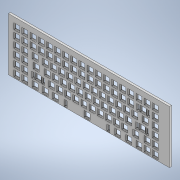
# Autodesk Inventor part: Top Plate
Saved by Autodesk Inventor 2020 (Build 240168000, 168)
## iProperties
Created: 2019-09-30
Part Number: Top Plate
Material: Generic
Document SubType Name: Sheet Metal
Designer: risha
Density: 1 g/cm^3
Sheet Metal Rule: Default_mm
Appearance: Default
Author: risha
Autodesk Inventor part; units mm, degrees
(part 1 of 2)
ref_plane "YZ Plane" through (0, 0, 0) normal (1, 0, 0) x (0, 1, 0)
ref_plane "XZ Plane" through (0, 0, 0) normal (0, 1, 0) x (-1, 0, 0)
ref_plane "XY Plane" through (0, 0, 0) normal (0, 0, 1) x (1, 0, 0)
sketch "Sketch1" plane through (0, 0, 0) normal (0, 0, 1) x (1, 0, 0)
  line L0 (3.025, -2.525) -> (16.025, -2.525)
  line L1 (3.025, -16.525) -> (16.025, -16.525)
  line L2 (2.525, -3.025) -> (2.525, -16.025)
  line L3 (16.525, -3.025) -> (16.525, -16.025)
  arc A0 (3.025, -2.525) -> (2.525, -3.025) centre (3.025, -3.025) ccw
  arc A1 (16.525, -3.025) -> (16.025, -2.525) centre (16.025, -3.025) ccw
  arc A2 (2.525, -16.025) -> (3.025, -16.525) centre (3.025, -16.025) ccw
  arc A3 (16.025, -16.525) -> (16.525, -16.025) centre (16.025, -16.025) ccw
  line L4 (22.075, -2.525) -> (35.075, -2.525)
  line L5 (22.075, -16.525) -> (35.075, -16.525)
  line L6 (21.575, -3.025) -> (21.575, -16.025)
  line L7 (35.575, -3.025) -> (35.575, -16.025)
  arc A4 (22.075, -2.525) -> (21.575, -3.025) centre (22.075, -3.025) ccw
  arc A5 (35.575, -3.025) -> (35.075, -2.525) centre (35.075, -3.025) ccw
  arc A6 (21.575, -16.025) -> (22.075, -16.525) centre (22.075, -16.025) ccw
  arc A7 (35.075, -16.525) -> (35.575, -16.025) centre (35.075, -16.025) ccw
  line L8 (41.125, -2.525) -> (54.125, -2.525)
  line L9 (41.125, -16.525) -> (54.125, -16.525)
  line L10 (40.625, -3.025) -> (40.625, -16.025)
  line L11 (54.625, -3.025) -> (54.625, -16.025)
  arc A8 (41.125, -2.525) -> (40.625, -3.025) centre (41.125, -3.025) ccw
  arc A9 (54.625, -3.025) -> (54.125, -2.525) centre (54.125, -3.025) ccw
  arc A10 (40.625, -16.025) -> (41.125, -16.525) centre (41.125, -16.025) ccw
  arc A11 (54.125, -16.525) -> (54.625, -16.025) centre (54.125, -16.025) ccw
  line L12 (60.175, -2.525) -> (73.175, -2.525)
  line L13 (60.175, -16.525) -> (73.175, -16.525)
  line L14 (59.675, -3.025) -> (59.675, -16.025)
  line L15 (73.675, -3.025) -> (73.675, -16.025)
  arc A12 (60.175, -2.525) -> (59.675, -3.025) centre (60.175, -3.025) ccw
  arc A13 (73.675, -3.025) -> (73.175, -2.525) centre (73.175, -3.025) ccw
  arc A14 (59.675, -16.025) -> (60.175, -16.525) centre (60.175, -16.025) ccw
  arc A15 (73.175, -16.525) -> (73.675, -16.025) centre (73.175, -16.025) ccw
  line L16 (79.225, -2.525) -> (92.225, -2.525)
  line L17 (79.225, -16.525) -> (92.225, -16.525)
  line L18 (78.725, -3.025) -> (78.725, -16.025)
  line L19 (92.725, -3.025) -> (92.725, -16.025)
  arc A16 (79.225, -2.525) -> (78.725, -3.025) centre (79.225, -3.025) ccw
  arc A17 (92.725, -3.025) -> (92.225, -2.525) centre (92.225, -3.025) ccw
  arc A18 (78.725, -16.025) -> (79.225, -16.525) centre (79.225, -16.025) ccw
  arc A19 (92.225, -16.525) -> (92.725, -16.025) centre (92.225, -16.025) ccw
  line L20 (98.275, -2.525) -> (111.275, -2.525)
  line L21 (98.275, -16.525) -> (111.275, -16.525)
  line L22 (97.775, -3.025) -> (97.775, -16.025)
  line L23 (111.775, -3.025) -> (111.775, -16.025)
  arc A20 (98.275, -2.525) -> (97.775, -3.025) centre (98.275, -3.025) ccw
  arc A21 (111.775, -3.025) -> (111.275, -2.525) centre (111.275, -3.025) ccw
  arc A22 (97.775, -16.025) -> (98.275, -16.525) centre (98.275, -16.025) ccw
  arc A23 (111.275, -16.525) -> (111.775, -16.025) centre (111.275, -16.025) ccw
  line L24 (117.325, -2.525) -> (130.325, -2.525)
  line L25 (117.325, -16.525) -> (130.325, -16.525)
  line L26 (116.825, -3.025) -> (116.825, -16.025)
  line L27 (130.825, -3.025) -> (130.825, -16.025)
  arc A24 (117.325, -2.525) -> (116.825, -3.025) centre (117.325, -3.025) ccw
  arc A25 (130.825, -3.025) -> (130.325, -2.525) centre (130.325, -3.025) ccw
  arc A26 (116.825, -16.025) -> (117.325, -16.525) centre (117.325, -16.025) ccw
  arc A27 (130.325, -16.525) -> (130.825, -16.025) centre (130.325, -16.025) ccw
  line L28 (136.375, -2.525) -> (149.375, -2.525)
  line L29 (136.375, -16.525) -> (149.375, -16.525)
  line L30 (135.875, -3.025) -> (135.875, -16.025)
  line L31 (149.875, -3.025) -> (149.875, -16.025)
  arc A28 (136.375, -2.525) -> (135.875, -3.025) centre (136.375, -3.025) ccw
  arc A29 (149.875, -3.025) -> (149.375, -2.525) centre (149.375, -3.025) ccw
  arc A30 (135.875, -16.025) -> (136.375, -16.525) centre (136.375, -16.025) ccw
  arc A31 (149.375, -16.525) -> (149.875, -16.025) centre (149.375, -16.025) ccw
  line L32 (155.425, -2.525) -> (168.425, -2.525)
  line L33 (155.425, -16.525) -> (168.425, -16.525)
  line L34 (154.925, -3.025) -> (154.925, -16.025)
  line L35 (168.925, -3.025) -> (168.925, -16.025)
  arc A32 (155.425, -2.525) -> (154.925, -3.025) centre (155.425, -3.025) ccw
  arc A33 (168.925, -3.025) -> (168.425, -2.525) centre (168.425, -3.025) ccw
  arc A34 (154.925, -16.025) -> (155.425, -16.525) centre (155.425, -16.025) ccw
  arc A35 (168.425, -16.525) -> (168.925, -16.025) centre (168.425, -16.025) ccw
  line L36 (174.475, -2.525) -> (187.475, -2.525)
  line L37 (174.475, -16.525) -> (187.475, -16.525)
  line L38 (173.975, -3.025) -> (173.975, -16.025)
  line L39 (187.975, -3.025) -> (187.975, -16.025)
  arc A36 (174.475, -2.525) -> (173.975, -3.025) centre (174.475, -3.025) ccw
  arc A37 (187.975, -3.025) -> (187.475, -2.525) centre (187.475, -3.025) ccw
  arc A38 (173.975, -16.025) -> (174.475, -16.525) centre (174.475, -16.025) ccw
  arc A39 (187.475, -16.525) -> (187.975, -16.025) centre (187.475, -16.025) ccw
  line L40 (193.525, -2.525) -> (206.525, -2.525)
  line L41 (193.525, -16.525) -> (206.525, -16.525)
  line L42 (193.025, -3.025) -> (193.025, -16.025)
  line L43 (207.025, -3.025) -> (207.025, -16.025)
  arc A40 (193.525, -2.525) -> (193.025, -3.025) centre (193.525, -3.025) ccw
  arc A41 (207.025, -3.025) -> (206.525, -2.525) centre (206.525, -3.025) ccw
  arc A42 (193.025, -16.025) -> (193.525, -16.525) centre (193.525, -16.025) ccw
  arc A43 (206.525, -16.525) -> (207.025, -16.025) centre (206.525, -16.025) ccw
  line L44 (212.575, -2.525) -> (225.575, -2.525)
  line L45 (212.575, -16.525) -> (225.575, -16.525)
  line L46 (212.075, -3.025) -> (212.075, -16.025)
  line L47 (226.075, -3.025) -> (226.075, -16.025)
  arc A44 (212.575, -2.525) -> (212.075, -3.025) centre (212.575, -3.025) ccw
  arc A45 (226.075, -3.025) -> (225.575, -2.525) centre (225.575, -3.025) ccw
  arc A46 (212.075, -16.025) -> (212.575, -16.525) centre (212.575, -16.025) ccw
  arc A47 (225.575, -16.525) -> (226.075, -16.025) centre (225.575, -16.025) ccw
  line L48 (231.625, -2.525) -> (244.625, -2.525)
  line L49 (231.625, -16.525) -> (244.625, -16.525)
  line L50 (231.125, -3.025) -> (231.125, -16.025)
  line L51 (245.125, -3.025) -> (245.125, -16.025)
  arc A48 (231.625, -2.525) -> (231.125, -3.025) centre (231.625, -3.025) ccw
  arc A49 (245.125, -3.025) -> (244.625, -2.525) centre (244.625, -3.025) ccw
  arc A50 (231.125, -16.025) -> (231.625, -16.525) centre (231.625, -16.025) ccw
  arc A51 (244.625, -16.525) -> (245.125, -16.025) centre (244.625, -16.025) ccw
  line L52 (250.675, -2.525) -> (263.675, -2.525)
  line L53 (250.675, -16.525) -> (263.675, -16.525)
  line L54 (250.175, -3.025) -> (250.175, -16.025)
  line L55 (264.175, -3.025) -> (264.175, -16.025)
  arc A52 (250.675, -2.525) -> (250.175, -3.025) centre (250.675, -3.025) ccw
  arc A53 (264.175, -3.025) -> (263.675, -2.525) centre (263.675, -3.025) ccw
  arc A54 (250.175, -16.025) -> (250.675, -16.525) centre (250.675, -16.025) ccw
  arc A55 (263.675, -16.525) -> (264.175, -16.025) centre (263.675, -16.025) ccw
  line L56 (269.725, -2.525) -> (282.725, -2.525)
  line L57 (269.725, -16.525) -> (282.725, -16.525)
  line L58 (269.225, -3.025) -> (269.225, -16.025)
  line L59 (283.225, -3.025) -> (283.225, -16.025)
  arc A56 (269.725, -2.525) -> (269.225, -3.025) centre (269.725, -3.025) ccw
  arc A57 (283.225, -3.025) -> (282.725, -2.525) centre (282.725, -3.025) ccw
  arc A58 (269.225, -16.025) -> (269.725, -16.525) centre (269.725, -16.025) ccw
  arc A59 (282.725, -16.525) -> (283.225, -16.025) centre (282.725, -16.025) ccw
  line L60 (288.775, -2.525) -> (301.775, -2.525)
  line L61 (288.775, -16.525) -> (301.775, -16.525)
  line L62 (288.275, -3.025) -> (288.275, -16.025)
  line L63 (302.275, -3.025) -> (302.275, -16.025)
  arc A60 (288.775, -2.525) -> (288.275, -3.025) centre (288.775, -3.025) ccw
  arc A61 (302.275, -3.025) -> (301.775, -2.525) centre (301.775, -3.025) ccw
  arc A62 (288.275, -16.025) -> (288.775, -16.525) centre (288.775, -16.025) ccw
  arc A63 (301.775, -16.525) -> (302.275, -16.025) centre (301.775, -16.025) ccw
  line L64 (307.825, -2.525) -> (320.825, -2.525)
  line L65 (307.825, -16.525) -> (320.825, -16.525)
  line L66 (307.325, -3.025) -> (307.325, -16.025)
  line L67 (321.325, -3.025) -> (321.325, -16.025)
  arc A64 (307.825, -2.525) -> (307.325, -3.025) centre (307.825, -3.025) ccw
  arc A65 (321.325, -3.025) -> (320.825, -2.525) centre (320.825, -3.025) ccw
  arc A66 (307.325, -16.025) -> (307.825, -16.525) centre (307.825, -16.025) ccw
  arc A67 (320.825, -16.525) -> (321.325, -16.025) centre (320.825, -16.025) ccw
  line L68 (326.875, -2.525) -> (339.875, -2.525)
  line L69 (326.875, -16.525) -> (339.875, -16.525)
  line L70 (326.375, -3.025) -> (326.375, -16.025)
  line L71 (340.375, -3.025) -> (340.375, -16.025)
  arc A68 (326.875, -2.525) -> (326.375, -3.025) centre (326.875, -3.025) ccw
  arc A69 (340.375, -3.025) -> (339.875, -2.525) centre (339.875, -3.025) ccw
  arc A70 (326.375, -16.025) -> (326.875, -16.525) centre (326.875, -16.025) ccw
  arc A71 (339.875, -16.525) -> (340.375, -16.025) centre (339.875, -16.025) ccw
  line L72 (3.025, -21.575) -> (16.025, -21.575)
  line L73 (3.025, -35.575) -> (16.025, -35.575)
  line L74 (2.525, -22.075) -> (2.525, -35.075)
  line L75 (16.525, -22.075) -> (16.525, -35.075)
  arc A72 (3.025, -21.575) -> (2.525, -22.075) centre (3.025, -22.075) ccw
  arc A73 (16.525, -22.075) -> (16.025, -21.575) centre (16.025, -22.075) ccw
  arc A74 (2.525, -35.075) -> (3.025, -35.575) centre (3.025, -35.075) ccw
  arc A75 (16.025, -35.575) -> (16.525, -35.075) centre (16.025, -35.075) ccw
  line L76 (22.075, -21.575) -> (35.075, -21.575)
  line L77 (22.075, -35.575) -> (35.075, -35.575)
  line L78 (21.575, -22.075) -> (21.575, -35.075)
  line L79 (35.575, -22.075) -> (35.575, -35.075)
  arc A76 (22.075, -21.575) -> (21.575, -22.075) centre (22.075, -22.075) ccw
  arc A77 (35.575, -22.075) -> (35.075, -21.575) centre (35.075, -22.075) ccw
  arc A78 (21.575, -35.075) -> (22.075, -35.575) centre (22.075, -35.075) ccw
  arc A79 (35.075, -35.575) -> (35.575, -35.075) centre (35.075, -35.075) ccw
  line L80 (41.125, -21.575) -> (54.125, -21.575)
  line L81 (41.125, -35.575) -> (54.125, -35.575)
  line L82 (40.625, -22.075) -> (40.625, -35.075)
  line L83 (54.625, -22.075) -> (54.625, -35.075)
  arc A80 (41.125, -21.575) -> (40.625, -22.075) centre (41.125, -22.075) ccw
  arc A81 (54.625, -22.075) -> (54.125, -21.575) centre (54.125, -22.075) ccw
  arc A82 (40.625, -35.075) -> (41.125, -35.575) centre (41.125, -35.075) ccw
  arc A83 (54.125, -35.575) -> (54.625, -35.075) centre (54.125, -35.075) ccw
  line L84 (60.175, -21.575) -> (73.175, -21.575)
  line L85 (60.175, -35.575) -> (73.175, -35.575)
  line L86 (59.675, -22.075) -> (59.675, -35.075)
  line L87 (73.675, -22.075) -> (73.675, -35.075)
  arc A84 (60.175, -21.575) -> (59.675, -22.075) centre (60.175, -22.075) ccw
  arc A85 (73.675, -22.075) -> (73.175, -21.575) centre (73.175, -22.075) ccw
  arc A86 (59.675, -35.075) -> (60.175, -35.575) centre (60.175, -35.075) ccw
  arc A87 (73.175, -35.575) -> (73.675, -35.075) centre (73.175, -35.075) ccw
  line L88 (79.225, -21.575) -> (92.225, -21.575)
  line L89 (79.225, -35.575) -> (92.225, -35.575)
  line L90 (78.725, -22.075) -> (78.725, -35.075)
  line L91 (92.725, -22.075) -> (92.725, -35.075)
  arc A88 (79.225, -21.575) -> (78.725, -22.075) centre (79.225, -22.075) ccw
  arc A89 (92.725, -22.075) -> (92.225, -21.575) centre (92.225, -22.075) ccw
  arc A90 (78.725, -35.075) -> (79.225, -35.575) centre (79.225, -35.075) ccw
  arc A91 (92.225, -35.575) -> (92.725, -35.075) centre (92.225, -35.075) ccw
  line L92 (98.275, -21.575) -> (111.275, -21.575)
  line L93 (98.275, -35.575) -> (111.275, -35.575)
  line L94 (97.775, -22.075) -> (97.775, -35.075)
  line L95 (111.775, -22.075) -> (111.775, -35.075)
  arc A92 (98.275, -21.575) -> (97.775, -22.075) centre (98.275, -22.075) ccw
  arc A93 (111.775, -22.075) -> (111.275, -21.575) centre (111.275, -22.075) ccw
  arc A94 (97.775, -35.075) -> (98.275, -35.575) centre (98.275, -35.075) ccw
  arc A95 (111.275, -35.575) -> (111.775, -35.075) centre (111.275, -35.075) ccw
  line L96 (117.325, -21.575) -> (130.325, -21.575)
  line L97 (117.325, -35.575) -> (130.325, -35.575)
  line L98 (116.825, -22.075) -> (116.825, -35.075)
  line L99 (130.825, -22.075) -> (130.825, -35.075)
  arc A96 (117.325, -21.575) -> (116.825, -22.075) centre (117.325, -22.075) ccw
  arc A97 (130.825, -22.075) -> (130.325, -21.575) centre (130.325, -22.075) ccw
  arc A98 (116.825, -35.075) -> (117.325, -35.575) centre (117.325, -35.075) ccw
  arc A99 (130.325, -35.575) -> (130.825, -35.075) centre (130.325, -35.075) ccw
  line L100 (136.375, -21.575) -> (149.375, -21.575)
  line L101 (136.375, -35.575) -> (149.375, -35.575)
  line L102 (135.875, -22.075) -> (135.875, -35.075)
  line L103 (149.875, -22.075) -> (149.875, -35.075)
  arc A100 (136.375, -21.575) -> (135.875, -22.075) centre (136.375, -22.075) ccw
  arc A101 (149.875, -22.075) -> (149.375, -21.575) centre (149.375, -22.075) ccw
  arc A102 (135.875, -35.075) -> (136.375, -35.575) centre (136.375, -35.075) ccw
  arc A103 (149.375, -35.575) -> (149.875, -35.075) centre (149.375, -35.075) ccw
  line L104 (155.425, -21.575) -> (168.425, -21.575)
  line L105 (155.425, -35.575) -> (168.425, -35.575)
  line L106 (154.925, -22.075) -> (154.925, -35.075)
  line L107 (168.925, -22.075) -> (168.925, -35.075)
  arc A104 (155.425, -21.575) -> (154.925, -22.075) centre (155.425, -22.075) ccw
  arc A105 (168.925, -22.075) -> (168.425, -21.575) centre (168.425, -22.075) ccw
  arc A106 (154.925, -35.075) -> (155.425, -35.575) centre (155.425, -35.075) ccw
  arc A107 (168.425, -35.575) -> (168.925, -35.075) centre (168.425, -35.075) ccw
  line L108 (174.475, -21.575) -> (187.475, -21.575)
  line L109 (174.475, -35.575) -> (187.475, -35.575)
  line L110 (173.975, -22.075) -> (173.975, -35.075)
  line L111 (187.975, -22.075) -> (187.975, -35.075)
  arc A108 (174.475, -21.575) -> (173.975, -22.075) centre (174.475, -22.075) ccw
  arc A109 (187.975, -22.075) -> (187.475, -21.575) centre (187.475, -22.075) ccw
  arc A110 (173.975, -35.075) -> (174.475, -35.575) centre (174.475, -35.075) ccw
  arc A111 (187.475, -35.575) -> (187.975, -35.075) centre (187.475, -35.075) ccw
  line L112 (193.525, -21.575) -> (206.525, -21.575)
  line L113 (193.525, -35.575) -> (206.525, -35.575)
  line L114 (193.025, -22.075) -> (193.025, -35.075)
  line L115 (207.025, -22.075) -> (207.025, -35.075)
  arc A112 (193.525, -21.575) -> (193.025, -22.075) centre (193.525, -22.075) ccw
  arc A113 (207.025, -22.075) -> (206.525, -21.575) centre (206.525, -22.075) ccw
  arc A114 (193.025, -35.075) -> (193.525, -35.575) centre (193.525, -35.075) ccw
  arc A115 (206.525, -35.575) -> (207.025, -35.075) centre (206.525, -35.075) ccw
  line L116 (212.575, -21.575) -> (225.575, -21.575)
  line L117 (212.575, -35.575) -> (225.575, -35.575)
  line L118 (212.075, -22.075) -> (212.075, -35.075)
  line L119 (226.075, -22.075) -> (226.075, -35.075)
  arc A116 (212.575, -21.575) -> (212.075, -22.075) centre (212.575, -22.075) ccw
  arc A117 (226.075, -22.075) -> (225.575, -21.575) centre (225.575, -22.075) ccw
  arc A118 (212.075, -35.075) -> (212.575, -35.575) centre (212.575, -35.075) ccw
  arc A119 (225.575, -35.575) -> (226.075, -35.075) centre (225.575, -35.075) ccw
  line L120 (231.625, -21.575) -> (244.625, -21.575)
  line L121 (231.625, -35.575) -> (244.625, -35.575)
  line L122 (231.125, -22.075) -> (231.125, -35.075)
  line L123 (245.125, -22.075) -> (245.125, -35.075)
  arc A120 (231.625, -21.575) -> (231.125, -22.075) centre (231.625, -22.075) ccw
  arc A121 (245.125, -22.075) -> (244.625, -21.575) centre (244.625, -22.075) ccw
  arc A122 (231.125, -35.075) -> (231.625, -35.575) centre (231.625, -35.075) ccw
  arc A123 (244.625, -35.575) -> (245.125, -35.075) centre (244.625, -35.075) ccw
  line L124 (250.675, -21.575) -> (263.675, -21.575)
  line L125 (250.675, -35.575) -> (263.675, -35.575)
  line L126 (250.175, -22.075) -> (250.175, -35.075)
  line L127 (264.175, -22.075) -> (264.175, -35.075)
  arc A124 (250.675, -21.575) -> (250.175, -22.075) centre (250.675, -22.075) ccw
  arc A125 (264.175, -22.075) -> (263.675, -21.575) centre (263.675, -22.075) ccw
  arc A126 (250.175, -35.075) -> (250.675, -35.575) centre (250.675, -35.075) ccw
  arc A127 (263.675, -35.575) -> (264.175, -35.075) centre (263.675, -35.075) ccw
  line L128 (269.725, -21.575) -> (282.725, -21.575)
  line L129 (269.725, -35.575) -> (282.725, -35.575)
  line L130 (269.225, -22.075) -> (269.225, -35.075)
  line L131 (283.225, -22.075) -> (283.225, -35.075)
  arc A128 (269.725, -21.575) -> (269.225, -22.075) centre (269.725, -22.075) ccw
  arc A129 (283.225, -22.075) -> (282.725, -21.575) centre (282.725, -22.075) ccw
  arc A130 (269.225, -35.075) -> (269.725, -35.575) centre (269.725, -35.075) ccw
  arc A131 (282.725, -35.575) -> (283.225, -35.075) centre (282.725, -35.075) ccw
  line L132 (298.3, -21.575) -> (311.3, -21.575)
  line L133 (298.3, -35.575) -> (311.3, -35.575)
  line L134 (297.8, -22.075) -> (297.8, -35.075)
  line L135 (311.8, -22.075) -> (311.8, -35.075)
  arc A132 (298.3, -21.575) -> (297.8, -22.075) centre (298.3, -22.075) ccw
  arc A133 (311.8, -22.075) -> (311.3, -21.575) centre (311.3, -22.075) ccw
  arc A134 (297.8, -35.075) -> (298.3, -35.575) centre (298.3, -35.075) ccw
  arc A135 (311.3, -35.575) -> (311.8, -35.075) centre (311.3, -35.075) ccw
  line L136 (313.863, -22.575) -> (319.613, -22.575)
  line L137 (313.863, -36.575) -> (319.613, -36.575)
  line L138 (313.363, -23.075) -> (313.363, -36.075)
  line L139 (320.113, -23.075) -> (320.113, -36.075)
  arc A136 (313.863, -22.575) -> (313.363, -23.075) centre (313.863, -23.075) ccw
  arc A137 (320.113, -23.075) -> (319.613, -22.575) centre (319.613, -23.075) ccw
  arc A138 (313.363, -36.075) -> (313.863, -36.575) centre (313.863, -36.075) ccw
  arc A139 (319.613, -36.575) -> (320.113, -36.075) centre (319.613, -36.075) ccw
  line L140 (289.987, -22.575) -> (295.737, -22.575)
  line L141 (289.987, -36.575) -> (295.737, -36.575)
  line L142 (289.487, -23.075) -> (289.487, -36.075)
  line L143 (296.237, -23.075) -> (296.237, -36.075)
  arc A140 (289.987, -22.575) -> (289.487, -23.075) centre (289.987, -23.075) ccw
  arc A141 (296.237, -23.075) -> (295.737, -22.575) centre (295.737, -23.075) ccw
  arc A142 (289.487, -36.075) -> (289.987, -36.575) centre (289.987, -36.075) ccw
  arc A143 (295.737, -36.575) -> (296.237, -36.075) centre (295.737, -36.075) ccw
  line L144 (326.875, -21.575) -> (339.875, -21.575)
  line L145 (326.875, -35.575) -> (339.875, -35.575)
  line L146 (326.375, -22.075) -> (326.375, -35.075)
  line L147 (340.375, -22.075) -> (340.375, -35.075)
  arc A144 (326.875, -21.575) -> (326.375, -22.075) centre (326.875, -22.075) ccw
  arc A145 (340.375, -22.075) -> (339.875, -21.575) centre (339.875, -22.075) ccw
  arc A146 (326.375, -35.075) -> (326.875, -35.575) centre (326.875, -35.075) ccw
  arc A147 (339.875, -35.575) -> (340.375, -35.075) centre (339.875, -35.075) ccw
  line L148 (3.025, -40.625) -> (16.025, -40.625)
  line L149 (3.025, -54.625) -> (16.025, -54.625)
  line L150 (2.525, -41.125) -> (2.525, -54.125)
  line L151 (16.525, -41.125) -> (16.525, -54.125)
  arc A148 (3.025, -40.625) -> (2.525, -41.125) centre (3.025, -41.125) ccw
  arc A149 (16.525, -41.125) -> (16.025, -40.625) centre (16.025, -41.125) ccw
  arc A150 (2.525, -54.125) -> (3.025, -54.625) centre (3.025, -54.125) ccw
  arc A151 (16.025, -54.625) -> (16.525, -54.125) centre (16.025, -54.125) ccw
  line L152 (22.075, -40.625) -> (35.075, -40.625)
  line L153 (22.075, -54.625) -> (35.075, -54.625)
  line L154 (21.575, -41.125) -> (21.575, -54.125)
  line L155 (35.575, -41.125) -> (35.575, -54.125)
  arc A152 (22.075, -40.625) -> (21.575, -41.125) centre (22.075, -41.125) ccw
  arc A153 (35.575, -41.125) -> (35.075, -40.625) centre (35.075, -41.125) ccw
  arc A154 (21.575, -54.125) -> (22.075, -54.625) centre (22.075, -54.125) ccw
  arc A155 (35.075, -54.625) -> (35.575, -54.125) centre (35.075, -54.125) ccw
  line L156 (45.8875, -40.625) -> (58.8875, -40.625)
  line L157 (45.8875, -54.625) -> (58.8875, -54.625)
  line L158 (45.3875, -41.125) -> (45.3875, -54.125)
  line L159 (59.3875, -41.125) -> (59.3875, -54.125)
  arc A156 (45.8875, -40.625) -> (45.3875, -41.125) centre (45.8875, -41.125) ccw
  arc A157 (59.3875, -41.125) -> (58.8875, -40.625) centre (58.8875, -41.125) ccw
  arc A158 (45.3875, -54.125) -> (45.8875, -54.625) centre (45.8875, -54.125) ccw
  arc A159 (58.8875, -54.625) -> (59.3875, -54.125) centre (58.8875, -54.125) ccw
  line L160 (69.7, -40.625) -> (82.7, -40.625)
  line L161 (69.7, -54.625) -> (82.7, -54.625)
  line L162 (69.2, -41.125) -> (69.2, -54.125)
  line L163 (83.2, -41.125) -> (83.2, -54.125)
  arc A160 (69.7, -40.625) -> (69.2, -41.125) centre (69.7, -41.125) ccw
  arc A161 (83.2, -41.125) -> (82.7, -40.625) centre (82.7, -41.125) ccw
  arc A162 (69.2, -54.125) -> (69.7, -54.625) centre (69.7, -54.125) ccw
  arc A163 (82.7, -54.625) -> (83.2, -54.125) centre (82.7, -54.125) ccw
  line L164 (88.75, -40.625) -> (101.75, -40.625)
  line L165 (88.75, -54.625) -> (101.75, -54.625)
  line L166 (88.25, -41.125) -> (88.25, -54.125)
  line L167 (102.25, -41.125) -> (102.25, -54.125)
  arc A164 (88.75, -40.625) -> (88.25, -41.125) centre (88.75, -41.125) ccw
  arc A165 (102.25, -41.125) -> (101.75, -40.625) centre (101.75, -41.125) ccw
  arc A166 (88.25, -54.125) -> (88.75, -54.625) centre (88.75, -54.125) ccw
  arc A167 (101.75, -54.625) -> (102.25, -54.125) centre (101.75, -54.125) ccw
  line L168 (107.8, -40.625) -> (120.8, -40.625)
  line L169 (107.8, -54.625) -> (120.8, -54.625)
  line L170 (107.3, -41.125) -> (107.3, -54.125)
  line L171 (121.3, -41.125) -> (121.3, -54.125)
  arc A168 (107.8, -40.625) -> (107.3, -41.125) centre (107.8, -41.125) ccw
  arc A169 (121.3, -41.125) -> (120.8, -40.625) centre (120.8, -41.125) ccw
  arc A170 (107.3, -54.125) -> (107.8, -54.625) centre (107.8, -54.125) ccw
  arc A171 (120.8, -54.625) -> (121.3, -54.125) centre (120.8, -54.125) ccw
  line L172 (126.85, -40.625) -> (139.85, -40.625)
  line L173 (126.85, -54.625) -> (139.85, -54.625)
  line L174 (126.35, -41.125) -> (126.35, -54.125)
  line L175 (140.35, -41.125) -> (140.35, -54.125)
  arc A172 (126.85, -40.625) -> (126.35, -41.125) centre (126.85, -41.125) ccw
  arc A173 (140.35, -41.125) -> (139.85, -40.625) centre (139.85, -41.125) ccw
  arc A174 (126.35, -54.125) -> (126.85, -54.625) centre (126.85, -54.125) ccw
  arc A175 (139.85, -54.625) -> (140.35, -54.125) centre (139.85, -54.125) ccw
  line L176 (145.9, -40.625) -> (158.9, -40.625)
  line L177 (145.9, -54.625) -> (158.9, -54.625)
  line L178 (145.4, -41.125) -> (145.4, -54.125)
  line L179 (159.4, -41.125) -> (159.4, -54.125)
  arc A176 (145.9, -40.625) -> (145.4, -41.125) centre (145.9, -41.125) ccw
  arc A177 (159.4, -41.125) -> (158.9, -40.625) centre (158.9, -41.125) ccw
  arc A178 (145.4, -54.125) -> (145.9, -54.625) centre (145.9, -54.125) ccw
  arc A179 (158.9, -54.625) -> (159.4, -54.125) centre (158.9, -54.125) ccw
  line L180 (164.95, -40.625) -> (177.95, -40.625)
  line L181 (164.95, -54.625) -> (177.95, -54.625)
  line L182 (164.45, -41.125) -> (164.45, -54.125)
  line L183 (178.45, -41.125) -> (178.45, -54.125)
  arc A180 (164.95, -40.625) -> (164.45, -41.125) centre (164.95, -41.125) ccw
  arc A181 (178.45, -41.125) -> (177.95, -40.625) centre (177.95, -41.125) ccw
  arc A182 (164.45, -54.125) -> (164.95, -54.625) centre (164.95, -54.125) ccw
  arc A183 (177.95, -54.625) -> (178.45, -54.125) centre (177.95, -54.125) ccw
  line L184 (184, -40.625) -> (197, -40.625)
  line L185 (184, -54.625) -> (197, -54.625)
  line L186 (183.5, -41.125) -> (183.5, -54.125)
  line L187 (197.5, -41.125) -> (197.5, -54.125)
  arc A184 (184, -40.625) -> (183.5, -41.125) centre (184, -41.125) ccw
  arc A185 (197.5, -41.125) -> (197, -40.625) centre (197, -41.125) ccw
  arc A186 (183.5, -54.125) -> (184, -54.625) centre (184, -54.125) ccw
  arc A187 (197, -54.625) -> (197.5, -54.125) centre (197, -54.125) ccw
  line L188 (203.05, -40.625) -> (216.05, -40.625)
  line L189 (203.05, -54.625) -> (216.05, -54.625)
  line L190 (202.55, -41.125) -> (202.55, -54.125)
  line L191 (216.55, -41.125) -> (216.55, -54.125)
  arc A188 (203.05, -40.625) -> (202.55, -41.125) centre (203.05, -41.125) ccw
  arc A189 (216.55, -41.125) -> (216.05, -40.625) centre (216.05, -41.125) ccw
  arc A190 (202.55, -54.125) -> (203.05, -54.625) centre (203.05, -54.125) ccw
  arc A191 (216.05, -54.625) -> (216.55, -54.125) centre (216.05, -54.125) ccw
  line L192 (222.1, -40.625) -> (235.1, -40.625)
  line L193 (222.1, -54.625) -> (235.1, -54.625)
  line L194 (221.6, -41.125) -> (221.6, -54.125)
  line L195 (235.6, -41.125) -> (235.6, -54.125)
  arc A192 (222.1, -40.625) -> (221.6, -41.125) centre (222.1, -41.125) ccw
  arc A193 (235.6, -41.125) -> (235.1, -40.625) centre (235.1, -41.125) ccw
  arc A194 (221.6, -54.125) -> (222.1, -54.625) centre (222.1, -54.125) ccw
  arc A195 (235.1, -54.625) -> (235.6, -54.125) centre (235.1, -54.125) ccw
  line L196 (241.15, -40.625) -> (254.15, -40.625)
  line L197 (241.15, -54.625) -> (254.15, -54.625)
  line L198 (240.65, -41.125) -> (240.65, -54.125)
  line L199 (254.65, -41.125) -> (254.65, -54.125)
  arc A196 (241.15, -40.625) -> (240.65, -41.125) centre (241.15, -41.125) ccw
  arc A197 (254.65, -41.125) -> (254.15, -40.625) centre (254.15, -41.125) ccw
  arc A198 (240.65, -54.125) -> (241.15, -54.625) centre (241.15, -54.125) ccw
  arc A199 (254.15, -54.625) -> (254.65, -54.125) centre (254.15, -54.125) ccw
  line L200 (260.2, -40.625) -> (273.2, -40.625)
  line L201 (260.2, -54.625) -> (273.2, -54.625)
  line L202 (259.7, -41.125) -> (259.7, -54.125)
  line L203 (273.7, -41.125) -> (273.7, -54.125)
  arc A200 (260.2, -40.625) -> (259.7, -41.125) centre (260.2, -41.125) ccw
  arc A201 (273.7, -41.125) -> (273.2, -40.625) centre (273.2, -41.125) ccw
  arc A202 (259.7, -54.125) -> (260.2, -54.625) centre (260.2, -54.125) ccw
  arc A203 (273.2, -54.625) -> (273.7, -54.125) centre (273.2, -54.125) ccw
  line L204 (279.25, -40.625) -> (292.25, -40.625)
  line L205 (279.25, -54.625) -> (292.25, -54.625)
  line L206 (278.75, -41.125) -> (278.75, -54.125)
  line L207 (292.75, -41.125) -> (292.75, -54.125)
  arc A204 (279.25, -40.625) -> (278.75, -41.125) centre (279.25, -41.125) ccw
  arc A205 (292.75, -41.125) -> (292.25, -40.625) centre (292.25, -41.125) ccw
  arc A206 (278.75, -54.125) -> (279.25, -54.625) centre (279.25, -54.125) ccw
  arc A207 (292.25, -54.625) -> (292.75, -54.125) centre (292.25, -54.125) ccw
  line L208 (303.0625, -40.625) -> (316.0625, -40.625)
  line L209 (303.0625, -54.625) -> (316.0625, -54.625)
  line L210 (302.5625, -41.125) -> (302.5625, -54.125)
  line L211 (316.5625, -41.125) -> (316.5625, -54.125)
  arc A208 (303.0625, -40.625) -> (302.5625, -41.125) centre (303.0625, -41.125) ccw
  arc A209 (316.5625, -41.125) -> (316.0625, -40.625) centre (316.0625, -41.125) ccw
  arc A210 (302.5625, -54.125) -> (303.0625, -54.625) centre (303.0625, -54.125) ccw
  arc A211 (316.0625, -54.625) -> (316.5625, -54.125) centre (316.0625, -54.125) ccw
  line L212 (326.875, -40.625) -> (339.875, -40.625)
  line L213 (326.875, -54.625) -> (339.875, -54.625)
  line L214 (326.375, -41.125) -> (326.375, -54.125)
  line L215 (340.375, -41.125) -> (340.375, -54.125)
  arc A212 (326.875, -40.625) -> (326.375, -41.125) centre (326.875, -41.125) ccw
  arc A213 (340.375, -41.125) -> (339.875, -40.625) centre (339.875, -41.125) ccw
  arc A214 (326.375, -54.125) -> (326.875, -54.625) centre (326.875, -54.125) ccw
  arc A215 (339.875, -54.625) -> (340.375, -54.125) centre (339.875, -54.125) ccw
  line L216 (3.025, -59.675) -> (16.025, -59.675)
  line L217 (3.025, -73.675) -> (16.025, -73.675)
  line L218 (2.525, -60.175) -> (2.525, -73.175)
  line L219 (16.525, -60.175) -> (16.525, -73.175)
  arc A216 (3.025, -59.675) -> (2.525, -60.175) centre (3.025, -60.175) ccw
  arc A217 (16.525, -60.175) -> (16.025, -59.675) centre (16.025, -60.175) ccw
  arc A218 (2.525, -73.175) -> (3.025, -73.675) centre (3.025, -73.175) ccw
  arc A219 (16.025, -73.675) -> (16.525, -73.175) centre (16.025, -73.175) ccw
  line L220 (22.075, -59.675) -> (35.075, -59.675)
  line L221 (22.075, -73.675) -> (35.075, -73.675)
  line L222 (21.575, -60.175) -> (21.575, -73.175)
  line L223 (35.575, -60.175) -> (35.575, -73.175)
  arc A220 (22.075, -59.675) -> (21.575, -60.175) centre (22.075, -60.175) ccw
  arc A221 (35.575, -60.175) -> (35.075, -59.675) centre (35.075, -60.175) ccw
  arc A222 (21.575, -73.175) -> (22.075, -73.675) centre (22.075, -73.175) ccw
  arc A223 (35.075, -73.675) -> (35.575, -73.175) centre (35.075, -73.175) ccw
  line L224 (48.2688, -59.675) -> (61.2687, -59.675)
  line L225 (48.2688, -73.675) -> (61.2687, -73.675)
  line L226 (47.7687, -60.175) -> (47.7687, -73.175)
  line L227 (61.7687, -60.175) -> (61.7687, -73.175)
  arc A224 (48.2688, -59.675) -> (47.7687, -60.175) centre (48.2688, -60.175) ccw
  arc A225 (61.7687, -60.175) -> (61.2687, -59.675) centre (61.2687, -60.175) ccw
  arc A226 (47.7687, -73.175) -> (48.2688, -73.675) centre (48.2688, -73.175) ccw
  arc A227 (61.2687, -73.675) -> (61.7687, -73.175) centre (61.2687, -73.175) ccw
  line L228 (74.4625, -59.675) -> (87.4625, -59.675)
  line L229 (74.4625, -73.675) -> (87.4625, -73.675)
  line L230 (73.9625, -60.175) -> (73.9625, -73.175)
  line L231 (87.9625, -60.175) -> (87.9625, -73.175)
  arc A228 (74.4625, -59.675) -> (73.9625, -60.175) centre (74.4625, -60.175) ccw
  arc A229 (87.9625, -60.175) -> (87.4625, -59.675) centre (87.4625, -60.175) ccw
  arc A230 (73.9625, -73.175) -> (74.4625, -73.675) centre (74.4625, -73.175) ccw
  arc A231 (87.4625, -73.675) -> (87.9625, -73.175) centre (87.4625, -73.175) ccw
  line L232 (93.5125, -59.675) -> (106.5125, -59.675)
  line L233 (93.5125, -73.675) -> (106.5125, -73.675)
  line L234 (93.0125, -60.175) -> (93.0125, -73.175)
  line L235 (107.0125, -60.175) -> (107.0125, -73.175)
  arc A232 (93.5125, -59.675) -> (93.0125, -60.175) centre (93.5125, -60.175) ccw
  arc A233 (107.0125, -60.175) -> (106.5125, -59.675) centre (106.5125, -60.175) ccw
  arc A234 (93.0125, -73.175) -> (93.5125, -73.675) centre (93.5125, -73.175) ccw
  arc A235 (106.5125, -73.675) -> (107.0125, -73.175) centre (106.5125, -73.175) ccw
  line L236 (112.5625, -59.675) -> (125.5625, -59.675)
  line L237 (112.5625, -73.675) -> (125.5625, -73.675)
  line L238 (112.0625, -60.175) -> (112.0625, -73.175)
  line L239 (126.0625, -60.175) -> (126.0625, -73.175)
  arc A236 (112.5625, -59.675) -> (112.0625, -60.175) centre (112.5625, -60.175) ccw
  arc A237 (126.0625, -60.175) -> (125.5625, -59.675) centre (125.5625, -60.175) ccw
  arc A238 (112.0625, -73.175) -> (112.5625, -73.675) centre (112.5625, -73.175) ccw
  arc A239 (125.5625, -73.675) -> (126.0625, -73.175) centre (125.5625, -73.175) ccw
  line L240 (131.6125, -59.675) -> (144.6125, -59.675)
  line L241 (131.6125, -73.675) -> (144.6125, -73.675)
  line L242 (131.1125, -60.175) -> (131.1125, -73.175)
  line L243 (145.1125, -60.175) -> (145.1125, -73.175)
  arc A240 (131.6125, -59.675) -> (131.1125, -60.175) centre (131.6125, -60.175) ccw
  arc A241 (145.1125, -60.175) -> (144.6125, -59.675) centre (144.6125, -60.175) ccw
  arc A242 (131.1125, -73.175) -> (131.6125, -73.675) centre (131.6125, -73.175) ccw
  arc A243 (144.6125, -73.675) -> (145.1125, -73.175) centre (144.6125, -73.175) ccw
  line L244 (150.6625, -59.675) -> (163.6625, -59.675)
  line L245 (150.6625, -73.675) -> (163.6625, -73.675)
  line L246 (150.1625, -60.175) -> (150.1625, -73.175)
  line L247 (164.1625, -60.175) -> (164.1625, -73.175)
  arc A244 (150.6625, -59.675) -> (150.1625, -60.175) centre (150.6625, -60.175) ccw
  arc A245 (164.1625, -60.175) -> (163.6625, -59.675) centre (163.6625, -60.175) ccw
  arc A246 (150.1625, -73.175) -> (150.6625, -73.675) centre (150.6625, -73.175) ccw
  arc A247 (163.6625, -73.675) -> (164.1625, -73.175) centre (163.6625, -73.175) ccw
  line L248 (169.7125, -59.675) -> (182.7125, -59.675)
  line L249 (169.7125, -73.675) -> (182.7125, -73.675)
  line L250 (169.2125, -60.175) -> (169.2125, -73.175)
  line L251 (183.2125, -60.175) -> (183.2125, -73.175)
  arc A248 (169.7125, -59.675) -> (169.2125, -60.175) centre (169.7125, -60.175) ccw
  arc A249 (183.2125, -60.175) -> (182.7125, -59.675) centre (182.7125, -60.175) ccw
  arc A250 (169.2125, -73.175) -> (169.7125, -73.675) centre (169.7125, -73.175) ccw
  arc A251 (182.7125, -73.675) -> (183.2125, -73.175) centre (182.7125, -73.175) ccw
  line L252 (188.7625, -59.675) -> (201.7625, -59.675)
  line L253 (188.7625, -73.675) -> (201.7625, -73.675)
  line L254 (188.2625, -60.175) -> (188.2625, -73.175)
  line L255 (202.2625, -60.175) -> (202.2625, -73.175)
  arc A252 (188.7625, -59.675) -> (188.2625, -60.175) centre (188.7625, -60.175) ccw
  arc A253 (202.2625, -60.175) -> (201.7625, -59.675) centre (201.7625, -60.175) ccw
  arc A254 (188.2625, -73.175) -> (188.7625, -73.675) centre (188.7625, -73.175) ccw
  arc A255 (201.7625, -73.675) -> (202.2625, -73.175) centre (201.7625, -73.175) ccw
  line L256 (207.8125, -59.675) -> (220.8125, -59.675)
  line L257 (207.8125, -73.675) -> (220.8125, -73.675)
  line L258 (207.3125, -60.175) -> (207.3125, -73.175)
  line L259 (221.3125, -60.175) -> (221.3125, -73.175)
  arc A256 (207.8125, -59.675) -> (207.3125, -60.175) centre (207.8125, -60.175) ccw
  arc A257 (221.3125, -60.175) -> (220.8125, -59.675) centre (220.8125, -60.175) ccw
  arc A258 (207.3125, -73.175) -> (207.8125, -73.675) centre (207.8125, -73.175) ccw
  arc A259 (220.8125, -73.675) -> (221.3125, -73.175) centre (220.8125, -73.175) ccw
  line L260 (226.8625, -59.675) -> (239.8625, -59.675)
  line L261 (226.8625, -73.675) -> (239.8625, -73.675)
  line L262 (226.3625, -60.175) -> (226.3625, -73.175)
  line L263 (240.3625, -60.175) -> (240.3625, -73.175)
  arc A260 (226.8625, -59.675) -> (226.3625, -60.175) centre (226.8625, -60.175) ccw
  arc A261 (240.3625, -60.175) -> (239.8625, -59.675) centre (239.8625, -60.175) ccw
  arc A262 (226.3625, -73.175) -> (226.8625, -73.675) centre (226.8625, -73.175) ccw
  arc A263 (239.8625, -73.675) -> (240.3625, -73.175) centre (239.8625, -73.175) ccw
  line L264 (245.9125, -59.675) -> (258.9125, -59.675)
  line L265 (245.9125, -73.675) -> (258.9125, -73.675)
  line L266 (245.4125, -60.175) -> (245.4125, -73.175)
  line L267 (259.4125, -60.175) -> (259.4125, -73.175)
  arc A264 (245.9125, -59.675) -> (245.4125, -60.175) centre (245.9125, -60.175) ccw
  arc A265 (259.4125, -60.175) -> (258.9125, -59.675) centre (258.9125, -60.175) ccw
  arc A266 (245.4125, -73.175) -> (245.9125, -73.675) centre (245.9125, -73.175) ccw
  arc A267 (258.9125, -73.675) -> (259.4125, -73.175) centre (258.9125, -73.175) ccw
  line L268 (264.9625, -59.675) -> (277.9625, -59.675)
  line L269 (264.9625, -73.675) -> (277.9625, -73.675)
  line L270 (264.4625, -60.175) -> (264.4625, -73.175)
  line L271 (278.4625, -60.175) -> (278.4625, -73.175)
  arc A268 (264.9625, -59.675) -> (264.4625, -60.175) centre (264.9625, -60.175) ccw
  arc A269 (278.4625, -60.175) -> (277.9625, -59.675) centre (277.9625, -60.175) ccw
  arc A270 (264.4625, -73.175) -> (264.9625, -73.675) centre (264.9625, -73.175) ccw
  arc A271 (277.9625, -73.675) -> (278.4625, -73.175) centre (277.9625, -73.175) ccw
  line L272 (295.9188, -59.675) -> (308.9187, -59.675)
  line L273 (295.9188, -73.675) -> (308.9187, -73.675)
  line L274 (295.4187, -60.175) -> (295.4187, -73.175)
  line L275 (309.4187, -60.175) -> (309.4187, -73.175)
  arc A272 (295.9188, -59.675) -> (295.4187, -60.175) centre (295.9188, -60.175) ccw
  arc A273 (309.4187, -60.175) -> (308.9187, -59.675) centre (308.9187, -60.175) ccw
  arc A274 (295.4187, -73.175) -> (295.9188, -73.675) centre (295.9188, -73.175) ccw
  arc A275 (308.9187, -73.675) -> (309.4187, -73.175) centre (308.9187, -73.175) ccw
  line L276 (311.4817, -60.675) -> (317.2317, -60.675)
  line L277 (311.4817, -74.675) -> (317.2317, -74.675)
  line L278 (310.9817, -61.175) -> (310.9817, -74.175)
  line L279 (317.7317, -61.175) -> (317.7317, -74.175)
  arc A276 (311.4817, -60.675) -> (310.9817, -61.175) centre (311.4817, -61.175) ccw
  arc A277 (317.7317, -61.175) -> (317.2317, -60.675) centre (317.2317, -61.175) ccw
  arc A278 (310.9817, -74.175) -> (311.4817, -74.675) centre (311.4817, -74.175) ccw
  arc A279 (317.2317, -74.675) -> (317.7317, -74.175) centre (317.2317, -74.175) ccw
  line L280 (287.6058, -60.675) -> (293.3558, -60.675)
  line L281 (287.6058, -74.675) -> (293.3558, -74.675)
  line L282 (287.1058, -61.175) -> (287.1058, -74.175)
  line L283 (293.8558, -61.175) -> (293.8558, -74.175)
  arc A280 (287.6058, -60.675) -> (287.1058, -61.175) centre (287.6058, -61.175) ccw
  arc A281 (293.8558, -61.175) -> (293.3558, -60.675) centre (293.3558, -61.175) ccw
  arc A282 (287.1058, -74.175) -> (287.6058, -74.675) centre (287.6058, -74.175) ccw
  arc A283 (293.3558, -74.675) -> (293.8558, -74.175) centre (293.3558, -74.175) ccw
  line L284 (326.875, -59.675) -> (339.875, -59.675)
  line L285 (326.875, -73.675) -> (339.875, -73.675)
  line L286 (326.375, -60.175) -> (326.375, -73.175)
  line L287 (340.375, -60.175) -> (340.375, -73.175)
  arc A284 (326.875, -59.675) -> (326.375, -60.175) centre (326.875, -60.175) ccw
  arc A285 (340.375, -60.175) -> (339.875, -59.675) centre (339.875, -60.175) ccw
  arc A286 (326.375, -73.175) -> (326.875, -73.675) centre (326.875, -73.175) ccw
  arc A287 (339.875, -73.675) -> (340.375, -73.175) centre (339.875, -73.175) ccw
  line L288 (3.025, -78.725) -> (16.025, -78.725)
  line L289 (3.025, -92.725) -> (16.025, -92.725)
  line L290 (2.525, -79.225) -> (2.525, -92.225)
  line L291 (16.525, -79.225) -> (16.525, -92.225)
  arc A288 (3.025, -78.725) -> (2.525, -79.225) centre (3.025, -79.225) ccw
  arc A289 (16.525, -79.225) -> (16.025, -78.725) centre (16.025, -79.225) ccw
  arc A290 (2.525, -92.225) -> (3.025, -92.725) centre (3.025, -92.225) ccw
  arc A291 (16.025, -92.725) -> (16.525, -92.225) centre (16.025, -92.225) ccw
  line L292 (22.075, -78.725) -> (35.075, -78.725)
  line L293 (22.075, -92.725) -> (35.075, -92.725)
  line L294 (21.575, -79.225) -> (21.575, -92.225)
  line L295 (35.575, -79.225) -> (35.575, -92.225)
  arc A292 (22.075, -78.725) -> (21.575, -79.225) centre (22.075, -79.225) ccw
  arc A293 (35.575, -79.225) -> (35.075, -78.725) centre (35.075, -79.225) ccw
  arc A294 (21.575, -92.225) -> (22.075, -92.725) centre (22.075, -92.225) ccw
  arc A295 (35.075, -92.725) -> (35.575, -92.225) centre (35.075, -92.225) ccw
  line L296 (53.0313, -78.725) -> (66.0312, -78.725)
  line L297 (53.0313, -92.725) -> (66.0312, -92.725)
  line L298 (52.5313, -79.225) -> (52.5313, -92.225)
  line L299 (66.5312, -79.225) -> (66.5312, -92.225)
  arc A296 (53.0313, -78.725) -> (52.5313, -79.225) centre (53.0313, -79.225) ccw
  arc A297 (66.5312, -79.225) -> (66.0312, -78.725) centre (66.0312, -79.225) ccw
  arc A298 (52.5313, -92.225) -> (53.0313, -92.725) centre (53.0313, -92.225) ccw
  arc A299 (66.0312, -92.725) -> (66.5312, -92.225) centre (66.0312, -92.225) ccw
  line L300 (68.5943, -79.725) -> (74.3443, -79.725)
  line L301 (68.5943, -93.725) -> (74.3443, -93.725)
  line L302 (68.0943, -80.225) -> (68.0943, -93.225)
  line L303 (74.8443, -80.225) -> (74.8443, -93.225)
  arc A300 (68.5943, -79.725) -> (68.0943, -80.225) centre (68.5943, -80.225) ccw
  arc A301 (74.8443, -80.225) -> (74.3443, -79.725) centre (74.3443, -80.225) ccw
  arc A302 (68.0943, -93.225) -> (68.5943, -93.725) centre (68.5943, -93.225) ccw
  arc A303 (74.3443, -93.725) -> (74.8443, -93.225) centre (74.3443, -93.225) ccw
  line L304 (44.7182, -79.725) -> (50.4682, -79.725)
  line L305 (44.7182, -93.725) -> (50.4682, -93.725)
  line L306 (44.2182, -80.225) -> (44.2182, -93.225)
  line L307 (50.9682, -80.225) -> (50.9682, -93.225)
  arc A304 (44.7182, -79.725) -> (44.2182, -80.225) centre (44.7182, -80.225) ccw
  arc A305 (50.9682, -80.225) -> (50.4682, -79.725) centre (50.4682, -80.225) ccw
  arc A306 (44.2182, -93.225) -> (44.7182, -93.725) centre (44.7182, -93.225) ccw
  arc A307 (50.4682, -93.725) -> (50.9682, -93.225) centre (50.4682, -93.225) ccw
  line L308 (83.9875, -78.725) -> (96.9875, -78.725)
  line L309 (83.9875, -92.725) -> (96.9875, -92.725)
  line L310 (83.4875, -79.225) -> (83.4875, -92.225)
  line L311 (97.4875, -79.225) -> (97.4875, -92.225)
  arc A308 (83.9875, -78.725) -> (83.4875, -79.225) centre (83.9875, -79.225) ccw
  arc A309 (97.4875, -79.225) -> (96.9875, -78.725) centre (96.9875, -79.225) ccw
  arc A310 (83.4875, -92.225) -> (83.9875, -92.725) centre (83.9875, -92.225) ccw
  arc A311 (96.9875, -92.725) -> (97.4875, -92.225) centre (96.9875, -92.225) ccw
  line L312 (103.0375, -78.725) -> (116.0375, -78.725)
  line L313 (103.0375, -92.725) -> (116.0375, -92.725)
  line L314 (102.5375, -79.225) -> (102.5375, -92.225)
  line L315 (116.5375, -79.225) -> (116.5375, -92.225)
  arc A312 (103.0375, -78.725) -> (102.5375, -79.225) centre (103.0375, -79.225) ccw
  arc A313 (116.5375, -79.225) -> (116.0375, -78.725) centre (116.0375, -79.225) ccw
  arc A314 (102.5375, -92.225) -> (103.0375, -92.725) centre (103.0375, -92.225) ccw
  arc A315 (116.0375, -92.725) -> (116.5375, -92.225) centre (116.0375, -92.225) ccw
  line L316 (122.0875, -78.725) -> (135.0875, -78.725)
  line L317 (122.0875, -92.725) -> (135.0875, -92.725)
  line L318 (121.5875, -79.225) -> (121.5875, -92.225)
  line L319 (135.5875, -79.225) -> (135.5875, -92.225)
  arc A316 (122.0875, -78.725) -> (121.5875, -79.225) centre (122.0875, -79.225) ccw
  arc A317 (135.5875, -79.225) -> (135.0875, -78.725) centre (135.0875, -79.225) ccw
  arc A318 (121.5875, -92.225) -> (122.0875, -92.725) centre (122.0875, -92.225) ccw
  arc A319 (135.0875, -92.725) -> (135.5875, -92.225) centre (135.0875, -92.225) ccw
  line L320 (141.1375, -78.725) -> (154.1375, -78.725)
  line L321 (141.1375, -92.725) -> (154.1375, -92.725)
  line L322 (140.6375, -79.225) -> (140.6375, -92.225)
  line L323 (154.6375, -79.225) -> (154.6375, -92.225)
  arc A320 (141.1375, -78.725) -> (140.6375, -79.225) centre (141.1375, -79.225) ccw
  arc A321 (154.6375, -79.225) -> (154.1375, -78.725) centre (154.1375, -79.225) ccw
  arc A322 (140.6375, -92.225) -> (141.1375, -92.725) centre (141.1375, -92.225) ccw
  arc A323 (154.1375, -92.725) -> (154.6375, -92.225) centre (154.1375, -92.225) ccw
  line L324 (160.1875, -78.725) -> (173.1875, -78.725)
  line L325 (160.1875, -92.725) -> (173.1875, -92.725)
  line L326 (159.6875, -79.225) -> (159.6875, -92.225)
  line L327 (173.6875, -79.225) -> (173.6875, -92.225)
  arc A324 (160.1875, -78.725) -> (159.6875, -79.225) centre (160.1875, -79.225) ccw
  arc A325 (173.6875, -79.225) -> (173.1875, -78.725) centre (173.1875, -79.225) ccw
  arc A326 (159.6875, -92.225) -> (160.1875, -92.725) centre (160.1875, -92.225) ccw
  arc A327 (173.1875, -92.725) -> (173.6875, -92.225) centre (173.1875, -92.225) ccw
  line L328 (179.2375, -78.725) -> (192.2375, -78.725)
  line L329 (179.2375, -92.725) -> (192.2375, -92.725)
  line L330 (178.7375, -79.225) -> (178.7375, -92.225)
  line L331 (192.7375, -79.225) -> (192.7375, -92.225)
  arc A328 (179.2375, -78.725) -> (178.7375, -79.225) centre (179.2375, -79.225) ccw
  arc A329 (192.7375, -79.225) -> (192.2375, -78.725) centre (192.2375, -79.225) ccw
  arc A330 (178.7375, -92.225) -> (179.2375, -92.725) centre (179.2375, -92.225) ccw
  arc A331 (192.2375, -92.725) -> (192.7375, -92.225) centre (192.2375, -92.225) ccw
  line L332 (198.2875, -78.725) -> (211.2875, -78.725)
  line L333 (198.2875, -92.725) -> (211.2875, -92.725)
  line L334 (197.7875, -79.225) -> (197.7875, -92.225)
  line L335 (211.7875, -79.225) -> (211.7875, -92.225)
  arc A332 (198.2875, -78.725) -> (197.7875, -79.225) centre (198.2875, -79.225) ccw
  arc A333 (211.7875, -79.225) -> (211.2875, -78.725) centre (211.2875, -79.225) ccw
  arc A334 (197.7875, -92.225) -> (198.2875, -92.725) centre (198.2875, -92.225) ccw
  arc A335 (211.2875, -92.725) -> (211.7875, -92.225) centre (211.2875, -92.225) ccw
  line L336 (217.3375, -78.725) -> (230.3375, -78.725)
  line L337 (217.3375, -92.725) -> (230.3375, -92.725)
  line L338 (216.8375, -79.225) -> (216.8375, -92.225)
  line L339 (230.8375, -79.225) -> (230.8375, -92.225)
  arc A336 (217.3375, -78.725) -> (216.8375, -79.225) centre (217.3375, -79.225) ccw
  arc A337 (230.8375, -79.225) -> (230.3375, -78.725) centre (230.3375, -79.225) ccw
  arc A338 (216.8375, -92.225) -> (217.3375, -92.725) centre (217.3375, -92.225) ccw
  arc A339 (230.3375, -92.725) -> (230.8375, -92.225) centre (230.3375, -92.225) ccw
  line L340 (236.3875, -78.725) -> (249.3875, -78.725)
  line L341 (236.3875, -92.725) -> (249.3875, -92.725)
  line L342 (235.8875, -79.225) -> (235.8875, -92.225)
  line L343 (249.8875, -79.225) -> (249.8875, -92.225)
  arc A340 (236.3875, -78.725) -> (235.8875, -79.225) centre (236.3875, -79.225) ccw
  arc A341 (249.8875, -79.225) -> (249.3875, -78.725) centre (249.3875, -79.225) ccw
  arc A342 (235.8875, -92.225) -> (236.3875, -92.725) centre (236.3875, -92.225) ccw
  arc A343 (249.3875, -92.725) -> (249.8875, -92.225) centre (249.3875, -92.225) ccw
  line L344 (255.4375, -78.725) -> (268.4375, -78.725)
  line L345 (255.4375, -92.725) -> (268.4375, -92.725)
  line L346 (254.9375, -79.225) -> (254.9375, -92.225)
  line L347 (268.9375, -79.225) -> (268.9375, -92.225)
  arc A344 (255.4375, -78.725) -> (254.9375, -79.225) centre (255.4375, -79.225) ccw
  arc A345 (268.9375, -79.225) -> (268.4375, -78.725) centre (268.4375, -79.225) ccw
  arc A346 (254.9375, -92.225) -> (255.4375, -92.725) centre (255.4375, -92.225) ccw
  arc A347 (268.4375, -92.725) -> (268.9375, -92.225) centre (268.4375, -92.225) ccw
  line L348 (281.6313, -78.725) -> (294.6313, -78.725)
  line L349 (281.6313, -92.725) -> (294.6313, -92.725)
  line L350 (281.1313, -79.225) -> (281.1313, -92.225)
  line L351 (295.1313, -79.225) -> (295.1313, -92.225)
  arc A348 (281.6313, -78.725) -> (281.1313, -79.225) centre (281.6313, -79.225) ccw
  arc A349 (295.1313, -79.225) -> (294.6313, -78.725) centre (294.6313, -79.225) ccw
  arc A350 (281.1313, -92.225) -> (281.6313, -92.725) centre (281.6313, -92.225) ccw
  arc A351 (294.6313, -92.725) -> (295.1313, -92.225) centre (294.6313, -92.225) ccw
  line L352 (307.825, -78.725) -> (320.825, -78.725)
  line L353 (307.825, -92.725) -> (320.825, -92.725)
  line L354 (307.325, -79.225) -> (307.325, -92.225)
  line L355 (321.325, -79.225) -> (321.325, -92.225)
  arc A352 (307.825, -78.725) -> (307.325, -79.225) centre (307.825, -79.225) ccw
  arc A353 (321.325, -79.225) -> (320.825, -78.725) centre (320.825, -79.225) ccw
  arc A354 (307.325, -92.225) -> (307.825, -92.725) centre (307.825, -92.225) ccw
  arc A355 (320.825, -92.725) -> (321.325, -92.225) centre (320.825, -92.225) ccw
  line L356 (326.875, -78.725) -> (339.875, -78.725)
  line L357 (326.875, -92.725) -> (339.875, -92.725)
  line L358 (326.375, -79.225) -> (326.375, -92.225)
  line L359 (340.375, -79.225) -> (340.375, -92.225)
  arc A356 (326.875, -78.725) -> (326.375, -79.225) centre (326.875, -79.225) ccw
  arc A357 (340.375, -79.225) -> (339.875, -78.725) centre (339.875, -79.225) ccw
  arc A358 (326.375, -92.225) -> (326.875, -92.725) centre (326.875, -92.225) ccw
  arc A359 (339.875, -92.725) -> (340.375, -92.225) centre (339.875, -92.225) ccw
  line L360 (3.025, -97.775) -> (16.025, -97.775)
  line L361 (3.025, -111.775) -> (16.025, -111.775)
  line L362 (2.525, -98.275) -> (2.525, -111.275)
  line L363 (16.525, -98.275) -> (16.525, -111.275)
  arc A360 (3.025, -97.775) -> (2.525, -98.275) centre (3.025, -98.275) ccw
  arc A361 (16.525, -98.275) -> (16.025, -97.775) centre (16.025, -98.275) ccw
  arc A362 (2.525, -111.275) -> (3.025, -111.775) centre (3.025, -111.275) ccw
  arc A363 (16.025, -111.775) -> (16.525, -111.275) centre (16.025, -111.275) ccw
  line L364 (22.075, -97.775) -> (35.075, -97.775)
  line L365 (22.075, -111.775) -> (35.075, -111.775)
  line L366 (21.575, -98.275) -> (21.575, -111.275)
  line L367 (35.575, -98.275) -> (35.575, -111.275)
  arc A364 (22.075, -97.775) -> (21.575, -98.275) centre (22.075, -98.275) ccw
  arc A365 (35.575, -98.275) -> (35.075, -97.775) centre (35.075, -98.275) ccw
  arc A366 (21.575, -111.275) -> (22.075, -111.775) centre (22.075, -111.275) ccw
  arc A367 (35.075, -111.775) -> (35.575, -111.275) centre (35.075, -111.275) ccw
  line L368 (45.8875, -97.775) -> (58.8875, -97.775)
  line L369 (45.8875, -111.775) -> (58.8875, -111.775)
  line L370 (45.3875, -98.275) -> (45.3875, -111.275)
  line L371 (59.3875, -98.275) -> (59.3875, -111.275)
  arc A368 (45.8875, -97.775) -> (45.3875, -98.275) centre (45.8875, -98.275) ccw
  arc A369 (59.3875, -98.275) -> (58.8875, -97.775) centre (58.8875, -98.275) ccw